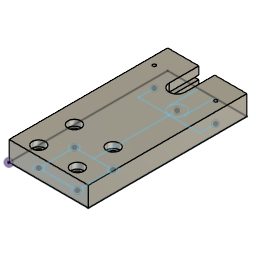
solenoid bracket v7 (Autodesk Fusion 360 design; units mm, degrees)
Autodesk Fusion 360 part; units mm, degrees
note: some values were not read from the file. Set by a fixed rule: which sketch regions a step uses.
sketch "Sketch1" plane through (0, 0, 0) normal (0, 0, 1) x (1, 0, 0)
  line L0 (0, 0) -> (40, 0)
  line L1 (40, 0) -> (40, 80)
  line L2 (40, 80) -> (0, 80)
  line L3 (0, 80) -> (0, 0)
  line L4 (10, 5) -> (29.5, 5)
  line L5 (29.5, 5) -> (29.5, 23)
  line L6 (29.5, 23) -> (10, 23)
  line L7 (10, 23) -> (10, 5)
  line L8 (19.75, 23) -> (19.75, 65)
  circle A0 centre (19.75, 65) radius 4
  circle A1 centre (10, 23) radius 2
  circle A2 centre (10, 5) radius 2
  circle A3 centre (29.5, 23) radius 2
  circle A4 centre (29.5, 5) radius 2
  line L9 (15.75, 65) -> (15.75, 80)
  line L10 (23.75, 65) -> (23.75, 80)
  line L11 (19.75, 61) -> (35.25, 61)
  line L12 (19.75, 61) -> (4.25, 61)
  line L13 (35.25, 61) -> (35.25, 69)
  circle A5 centre (35.25, 69) radius 0.8
  line L14 (4.25, 61) -> (4.25, 69)
  circle A6 centre (4.25, 69) radius 0.8
  dimension "d1" = 40
  dimension "d2" = 80
  dimension "d3" = 19.5
  dimension "d4" = 18
  dimension "d6" = 42
  dimension "d7" = 8
  dimension "d8" = 4
  dimension "d9" = 4
  dimension "d10" = 4
  dimension "d11" = 4
  dimension "d22" = 15.5
  dimension "d23" = 15.5
  dimension "d24" = 8
  dimension "d25" = 1.6
  dimension "d26" = 8
  dimension "d27" = 1.6
  constraint horizontal L0
  constraint vertical L1
  constraint horizontal L2
  constraint vertical L3
  constraint coincident L0.start L3.end
  constraint horizontal L4
  constraint vertical L5
  constraint horizontal L6
  constraint vertical L7
  constraint midpoint L6 L8.start
  constraint perpendicular L6 L8
  constraint coincident L8.end A0.centre
  constraint coincident L6.end L7.start
  constraint coincident L4.start L7.end
  constraint coincident L5.end L6.start
  constraint coincident L4.end L5.start
  constraint coincident A0 L9.start
  constraint coincident L2 L9.end
  constraint tangent A0 L9
  constraint perpendicular L2 L9
  constraint coincident A0 L10.start
  constraint coincident L2 L10.end
  constraint tangent A0 L10
  constraint perpendicular L2 L10
  constraint coincident A0 L11.start
  constraint coincident L8 L11.start
  constraint perpendicular L1 L11
  constraint perpendicular L8 L12
  constraint perpendicular L11 L13
  constraint coincident L13.end A5.centre
  constraint perpendicular L12 L14
  constraint coincident L14.end A6.centre
  measures "d1" distance of L0.start L0.end
  measures "d2" distance of L0.start L2.end
  measures "d3" distance of L4.start L4.end
  measures "d4" distance of L4.start L6.end
  measures "d6" distance of L8.start L8.end
  measures "d7" diameter of A0
  measures "d8" diameter of A1
  measures "d9" diameter of A2
  measures "d10" diameter of A3
  measures "d11" diameter of A4
  measures "d22" distance of L11.start L11.end
  measures "d23" distance of L11.start L12.end
  measures "d24" distance of L11.end L13.end
  measures "d25" diameter of A5
  measures "d26" distance of L12.end L14.end
  measures "d27" diameter of A6
extrude "Extrude1" add sketch "Sketch1" along normal blind 10 contours L0 L1 L2 L3 A0 L9 L10 | L4 L5 L6 L7 A1 A2 A3 A4
sketch "Sketch3" plane through (0, 80, 0) normal (0, 1, 0) x (-1, 0, 0)
  line L0 (-40, 0) -> (-23.75, 0)
  line L1 (-23.75, 0) -> (-23.75, 10)
  line L2 (-23.75, 10) -> (-40, 10)
  line L3 (-40, 10) -> (-40, 0)
  line L4 (-40, 0) -> (-40, 4)
  line L5 (-40, 4) -> (-40, 6)
  line L6 (-40, 6) -> (-40, 10)
  line L7 (-20, 4) -> (-20, 6)
  line L8 (-20, 5) -> (-1.25, 5)
  line L9 (-20, 5) -> (-38.75, 5)
  line L10 (-38.75, 5) -> (-38.75, 6)
  line L11 (-1.25, 5) -> (-1.25, 4)
  line L12 (-38.75, 6) -> (-1.25, 6)
  line L13 (-1.25, 6) -> (-1.25, 4)
  line L14 (-1.25, 4) -> (-38.75, 4)
  line L15 (-38.75, 4) -> (-38.75, 6)
  dimension "d14" = 4
  dimension "d15" = 2
  dimension "d16" = 18.75
  dimension "d17" = 18.75
  dimension "d18" = 1
  dimension "d19" = 1
  constraint coincident L0.start L3.end
  constraint perpendicular L0 L4
  constraint parallel L3 L5
  constraint coincident L2.end L3.start
  constraint midpoint L7 L8.start
  constraint perpendicular L7 L8
  constraint perpendicular L7 L9
  constraint perpendicular L9 L10
  constraint perpendicular L8 L11
  constraint horizontal L12
  constraint vertical L13
  constraint horizontal L14
  constraint vertical L15
  measures "d14" distance of L0.start L4.end
  measures "d15" distance of L4.end L5.end
  measures "d16" distance of L8.start L8.end
  measures "d17" distance of L8.start L9.end
  measures "d18" distance of L9.end L10.end
  measures "d19" distance of L8.end L11.end
extrude "Extrude2" cut sketch "Sketch3" against normal blind 31 contours L1 L9 L14 L15 | L1 L7 L9 L14 | L1 L9 L10 L12 L15 | L1 L7 L9 L12 | L7 L8 L11 L13 L14 | L7 L8 L12 L13
sketch "Sketch4" plane through (0, 49, 0) normal (0, 1, 0) x (-1, 0, 0)
  line L0 (-1.25, 6) -> (-38.75, 6)
  line L1 (-38.75, 6) -> (-38.75, 4)
  line L2 (-38.75, 4) -> (-1.25, 4)
  line L3 (-1.25, 4) -> (-1.25, 6)
  line L4 (-22.5, 6) -> (-17.5, 6)
  line L5 (-17.5, 6) -> (-17.5, 4)
  line L6 (-17.5, 4) -> (-22.5, 4)
  line L7 (-22.5, 4) -> (-22.5, 6)
  dimension "d30" = 5
  dimension "d31" = 2
  constraint horizontal L4
  constraint vertical L5
  constraint horizontal L6
  constraint vertical L7
  constraint coincident L0 L4.start
  measures "d30" distance of L4.start L4.end
  measures "d31" distance of L4.start L6.end
extrude "Extrude3" cut sketch "Sketch4" against normal blind 6 contours L0 L2 L4 L5 L6 L7
sketch "Sketch5" plane through (0, 0, 10) normal (0, 0, 1) x (-1, 0, 0)
  circle A0 centre (-10, -23) radius 2
  circle A1 centre (-29.5, -5) radius 2
  circle A2 centre (-35.25, -69) radius 0.8
  circle A3 centre (-4.25, -69) radius 0.8
  circle A4 centre (-29.5, -23) radius 2
  circle A5 centre (-10, -5) radius 2
  line L0 (-15.75, -65) -> (-15.75, -80)
  line L1 (-15.75, -80) -> (0, -80)
  line L2 (0, -80) -> (0, 0)
  line L3 (0, 0) -> (-40, 0)
  line L4 (-40, 0) -> (-40, -80)
  line L5 (-40, -80) -> (-23.75, -80)
  line L6 (-23.75, -80) -> (-23.75, -65)
  arc A6 (-15.75, -65) -> (-23.75, -65) centre (-19.75, -65) ccw
  circle A7 centre (-10, -5) radius 3.25
  circle A8 centre (-10, -23) radius 3.25
  circle A9 centre (-29.5, -5) radius 3.25
  circle A10 centre (-29.5, -23) radius 3.25
  dimension "d34" = 6.5
  dimension "d35" = 6.5
  dimension "d36" = 6.5
  dimension "d37" = 6.5
  constraint concentric A5 A7
  constraint concentric A0 A8
  constraint concentric A1 A9
  constraint concentric A4 A10
  measures "d34" diameter of A7
  measures "d35" diameter of A8
  measures "d36" diameter of A9
  measures "d37" diameter of A10
extrude "Extrude4" cut sketch "Sketch5" against normal blind 3 contours A7 | A8 | A9 | A10
